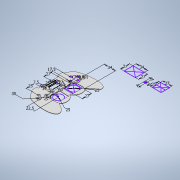
# Autodesk Inventor part: ovladac
Saved by Autodesk Inventor 2022 (Build 260153000, 153)
## iProperties
Created: 2022-12-02
Part Number: ovladac
Material: Generic
Document SubType Name: Modeling
Designer: matys
Density: 1 g/cm^3
Appearance: Default
Author: matys
Autodesk Inventor part; units mm, degrees
ref_plane "YZ Plane" through (0, 0, 0) normal (1, 0, 0) x (0, 1, 0)
ref_plane "XZ Plane" through (0, 0, 0) normal (0, 1, 0) x (-1, 0, 0)
ref_plane "XY Plane" through (0, 0, 0) normal (0, 0, 1) x (1, 0, 0)
sketch "Sketch1" plane through (0, 0, 0) normal (0, 1, 0) x (-1, 0, 0)
  circle A0 centre (0, 0) radius 17.5
  line L0 (0, -17.5) -> (0, -77.5)
  line L1 (0, -77.5) -> (0, -95)
  circle A1 centre (0, -95) radius 17.5
  line L2 (0, 0) -> (0, -25)
  line L3 (0, -25) -> (-22.5, -25)
  circle A2 centre (-22.5, -25) radius 12.5
  line L4 (-86.0476, -189.7218) -> (-86.0476, -216.7218)
  line L5 (-86.0476, -216.7218) -> (-52.0476, -216.7218)
  line L6 (-52.0476, -216.7218) -> (-52.0476, -189.7218)
  line L7 (-52.0476, -189.7218) -> (-86.0476, -189.7218)
  line L8 (-86.0476, -189.7218) -> (-52.0476, -216.7218)
  line L9 (-52.0476, -189.7218) -> (-86.0476, -216.7218)
  line L10 (0, -25) -> (0, -17.5)
  line L11 (0, -25) -> (0, -32.5)
  circle A3 centre (-22.5, -70) radius 12.5
  line L12 (-39.5, -56.5) -> (-39.5, -83.5)
  line L13 (-39.5, -83.5) -> (-5.5, -83.5)
  line L14 (-5.5, -83.5) -> (-5.5, -56.5)
  line L15 (-5.5, -56.5) -> (-39.5, -56.5)
  line L16 (-39.5, -56.5) -> (-5.5, -83.5)
  line L17 (-5.5, -56.5) -> (-39.5, -83.5)
  line L18 (-5.5, -56.5) -> (-22.5, -70)
  line L19 (-109.6323, -189.7218) -> (-115.6323, -189.7218)
  line L20 (-115.6323, -189.7218) -> (-115.6323, -195.7218)
  line L21 (-115.6323, -195.7218) -> (-109.6323, -195.7218)
  line L22 (-109.6323, -195.7218) -> (-109.6323, -189.7218)
  line L23 (-115.6323, -189.7218) -> (-109.6323, -195.7218)
  line L24 (-109.6323, -189.7218) -> (-115.6323, -195.7218)
  line L25 (0, -112.5) -> (0, -106)
  line L26 (-3, -109) -> (-3, -103)
  line L27 (-3, -103) -> (3, -103)
  line L28 (3, -103) -> (3, -109)
  line L29 (3, -109) -> (-3, -109)
  line L30 (14, -98) -> (8, -98)
  line L31 (14, -92) -> (14, -98)
  line L32 (8, -98) -> (8, -92)
  line L33 (8, -92) -> (14, -92)
  line L34 (3, -81) -> (3, -87)
  line L35 (-3, -81) -> (3, -81)
  line L36 (3, -87) -> (-3, -87)
  line L37 (-3, -87) -> (-3, -81)
  line L38 (-14, -92) -> (-8, -92)
  line L39 (-14, -98) -> (-14, -92)
  line L40 (-8, -92) -> (-8, -98)
  line L41 (-8, -98) -> (-14, -98)
  line L42 (-135.6088, -189.7218) -> (-135.6088, -214.7218)
  line L43 (-135.6088, -214.7218) -> (-162.6088, -214.7218)
  line L44 (-162.6088, -214.7218) -> (-162.6088, -189.7218)
  line L45 (-162.6088, -189.7218) -> (-135.6088, -189.7218)
  line L46 (-162.6088, -189.7218) -> (-135.6088, -214.7218)
  line L47 (-135.6088, -189.7218) -> (-162.6088, -214.7218)
  line L48 (17.5, 0) -> (17.5, -95)
  line L49 (-162.6088, -202.2218) -> (-135.6088, -202.2218)
  line L50 (25.5, -35) -> (25.5, -60)
  line L51 (25.5, -60) -> (-1.5, -60)
  line L52 (-1.5, -60) -> (-1.5, -35)
  line L53 (-1.5, -35) -> (25.5, -35)
  line L54 (25.5, -35) -> (20.5, -35)
  line L55 (20.5, -35) -> (20.5, -60)
  line L56 (-1.5, -35) -> (6.5, -35)
  line L57 (6.5, -35) -> (6.5, -60)
  line L58 (-1.5, -47.5) -> (6.5, -47.5)
  line L59 (-1.5, -35) -> (35.8, -35)
  line L60 (25.5, -60) -> (29.5, -60)
  line L61 (29.5, -60) -> (29.5, -47.5)
  line L62 (29.5, -47.5) -> (25.5, -47.5)
  line L63 (29.5, -60) -> (-7.8, -60)
  line L64 (-7.8, -60) -> (-7.8, -35)
  line L65 (-7.8, -35) -> (-1.5, -35)
  dimension "d0" = 35
  dimension "d1" = 60
  dimension "d2" = 17.5
  dimension "d3" = 25
  dimension "d4" = 22.5
  dimension "d6" = 25
  dimension "d7" = 27
  dimension "d8" = 34
  dimension "d9" = 27
  dimension "d10" = 7.5
  dimension "d11" = 25
  dimension "d12" = 27
  dimension "d13" = 34
  dimension "d14" = 27
  dimension "d15" = 6
  dimension "d16" = 6
  dimension "d17" = 6
  dimension "d18" = 6.5
  dimension "d22" = 6
  dimension "d25" = 360
  dimension "d27" = 25
  dimension "d28" = 27
  dimension "d32" = 25
  dimension "d33" = 27
  dimension "d34" = 5
  dimension "d35" = 8
  dimension "d36" = 8
  dimension "d72" = 37.3
  dimension "d73" = 4
  dimension "d74" = 37.3
  constraints: 132 end point, 20 perpendicular, 8 point on line, 8 vertical, 6 midpoint, 5 point on circle, 4 centre point, 3 coincident, 3 horizontal, 1 collinear, 1 tangent, 33 other
  measures "d0" diameter of A0
  measures "d1" distance of L0.start L0.end
  measures "d2" distance of L0.end L1.end
  measures "d3" distance of L2.start L2.end
  measures "d4" distance of L2.end L3.end
  measures "d6" diameter of A2
  measures "d7" distance of L4.start L4.end
  measures "d8" distance of L4.end L5.end
  measures "d9" distance of L5.end L6.end
  measures "d10" distance of L2.end L11.end
  measures "d11" diameter of A3
  measures "d12" distance of L15.end L12.end
  measures "d13" distance of L12.end L14.start
  measures "d14" distance of L14.start L15.start
  measures "d15" distance of L19.start L19.end
  measures "d16" distance of L19.end L20.end
  measures "d17" distance of L20.end L21.end
  measures "d18" distance of L25.start L25.end
  measures "d22" distance of L26.start L26.end
  measures "d27" distance of L42.start L42.end
  measures "d28" distance of L42.end L43.end
  measures "d32" distance of L50.start L50.end
  measures "d33" distance of L50.end L51.end
  measures "d34" distance of L50.start L54.end
  measures "d35" distance of L52.end L56.end
  measures "d36" distance between parallel lines of L50 L48
  measures "d72" distance of L52.end L59.end
  measures "d73" distance of L50.end L60.end
  measures "d74" distance of L60.end L63.end
sketch "Sketch2" plane through (0, 0, 0) normal (0, 1, 0) x (-1, 0, 0)
  circle A0 centre (0, 0) radius 17.5
  line L0 (0, 17.5) -> (0, 25.5)
  line L1 (17.5, 0) -> (29.5, 0)
  line L2 (0, 0) -> (0, 17.5)
  line L3 (0, 17.5) -> (17.5, 0)
  line L4 (0, 0) -> (8.75, 8.75)
  line L5 (8.75, 8.75) -> (12.3744, 12.3744)
  line L6 (12.3744, 12.3744) -> (18.0312, 18.0312)
  arc A1 (29.5, 0) -> (10.5727, 22.6518) centre (-3.4308, -8.2827) ccw
  line L7 (0, -20.5) -> (0, -80.5)
  line L8 (0, -80.5) -> (0, -98)
  line L9 (29.5, 0) -> (29.5, -17.5) construction
  line L10 (34.5, -12.5) -> (34.5, -5)
  arc A2 (34.5, -5) -> (29.5, 0) centre (29.5, -5) ccw
  arc A3 (29.5, -17.5) -> (34.5, -12.5) centre (29.5, -12.5) ccw
  line L11 (29.5, -17.5) -> (29.5, -47.5)
  line L12 (0, -20.5) -> (0, -25.5)
  line L13 (0, -17.5) -> (0, -21.5)
  ellipse E0 centre (-5.5218, 3.3783) end of major axis (-65.9225, 17.4065) minor radius 22.7978 (10.5727, 22.6518) -> (-28.0257, -13.7877) ccw
  line L14 (0, -17.5) -> (0, -25)
  line L15 (0, -25) -> (-22.5, -25)
  circle A4 centre (-22.5, -25) radius 12.5
  line L16 (-9, -8) -> (-36, -8)
  line L17 (-36, -8) -> (-36, -42)
  line L18 (-36, -42) -> (-9, -42)
  line L19 (-9, -42) -> (-9, -8)
  line L20 (-36, -42) -> (-9, -8)
  line L21 (-36, -8) -> (-9, -42)
  line L22 (-22.5, -25) -> (-36, -42)
  line L23 (0, -17.5) -> (0, -11)
  line L24 (0, -11) -> (3, -11)
  line L25 (3, -11) -> (3, -8)
  line L26 (3, -8) -> (-3, -8)
  line L27 (-3, -8) -> (-3, -14)
  line L28 (-3, -14) -> (3, -14)
  line L29 (3, -14) -> (3, -11)
  line L30 (14, 3) -> (11, 3)
  line L31 (8, 3) -> (8, -3)
  line L32 (11, 3) -> (8, 3)
  line L33 (8, -3) -> (14, -3)
  line L34 (14, -3) -> (14, 3)
  line L35 (-3, 14) -> (-3, 11)
  line L36 (-3, 8) -> (3, 8)
  line L37 (-3, 11) -> (-3, 8)
  line L38 (3, 8) -> (3, 14)
  line L39 (3, 14) -> (-3, 14)
  line L40 (-14, -3) -> (-11, -3)
  line L41 (-8, -3) -> (-8, 3)
  line L42 (-11, -3) -> (-8, -3)
  line L43 (-8, 3) -> (-14, 3)
  line L44 (-14, 3) -> (-14, -3)
  line L45 (0, -47.5) -> (-33.3972, -47.5)
  arc A5 (-41.1706, -8.3745) -> (-33.3972, -47.5) centre (-22.5, -25) ccw
  arc A6 (10.5727, -117.6518) -> (29.5, -95) centre (-3.4308, -86.7173) ccw
  line L46 (34.5, -82.5) -> (34.5, -90)
  arc A7 (29.5, -95) -> (34.5, -90) centre (29.5, -90) ccw
  arc A8 (34.5, -82.5) -> (29.5, -77.5) centre (29.5, -82.5) ccw
  line L47 (29.5, -77.5) -> (29.5, -47.5)
  ellipse E1 centre (-5.5218, -98.3783) end of major axis (-65.9225, -112.4065) minor radius 22.7978 (-28.0257, -81.2123) -> (10.5727, -117.6518) ccw
  arc A9 (-33.3972, -47.5) -> (-41.1706, -86.6255) centre (-22.5, -70) ccw
  line L48 (0, -95) -> (0, -112.5)
  line L49 (-9, -87) -> (-36, -87)
  line L50 (-36, -87) -> (-36, -53)
  line L51 (-36, -53) -> (-9, -53)
  line L52 (-9, -53) -> (-9, -87)
  line L53 (0, -77.5) -> (0, -84)
  line L54 (0, -84) -> (3, -84)
  line L55 (3, -84) -> (3, -87)
  line L56 (3, -87) -> (-3, -87)
  line L57 (-3, -87) -> (-3, -81)
  line L58 (-3, -81) -> (3, -81)
  line L59 (3, -81) -> (3, -84)
  line L60 (14, -98) -> (11, -98)
  line L61 (8, -98) -> (8, -92)
  line L62 (11, -98) -> (8, -98)
  line L63 (8, -92) -> (14, -92)
  line L64 (14, -92) -> (14, -98)
  line L65 (-3, -109) -> (-3, -106)
  line L66 (-3, -103) -> (3, -103)
  line L67 (-3, -106) -> (-3, -103)
  line L68 (3, -103) -> (3, -109)
  line L69 (3, -109) -> (-3, -109)
  line L70 (-14, -92) -> (-11, -92)
  line L71 (-8, -92) -> (-8, -98)
  line L72 (-11, -92) -> (-8, -92)
  line L73 (-8, -98) -> (-14, -98)
  line L74 (-14, -98) -> (-14, -92)
  line L75 (0, -47.5) -> (-1.5, -47.5)
  line L76 (-1.5, -47.5) -> (-1.5, -60)
  line L77 (-1.5, -60) -> (25.5, -60)
  line L78 (25.5, -60) -> (25.5, -35)
  line L79 (25.5, -35) -> (-1.5, -35)
  line L80 (-1.5, -35) -> (-1.5, -47.5)
  line L81 (0, -17.5) -> (0, -25)
  line L82 (0, -47.5) -> (0, -35)
  line L83 (25.5, -44.7664) -> (24.099, -44.7664)
  line L84 (-5.5218, 3.3783) -> (-65.9225, 17.4065)
  line L85 (-5.5218, 3.3783) -> (-5.5218, 9.5)
  line L86 (-65.9225, 17.4065) -> (128.8922, -27.8397)
  point P0 (29.5, -8.75)
  point P1 (0, -35)
  point P2 (0, -60)
  dimension "d50" = 25
  dimension "d37" = 35
  dimension "d38" = 8
  dimension "d39" = 12
  dimension "d40" = 8
  dimension "d41" = 60
  dimension "d42" = 17.5
  dimension "d47" = 4
  dimension "d48" = 7.5
  dimension "d49" = 22.5
  dimension "d51" = 27
  dimension "d52" = 34
  dimension "d53" = 6.5
  dimension "d54" = 3
  dimension "d55" = 3
  dimension "d56" = 6
  dimension "d57" = 6
  dimension "d60" = 360
  dimension "d65" = 1.5
  dimension "d66" = 12.5
  dimension "d67" = 27
  dimension "d68" = 25
  dimension "d69" = 1.401
  dimension "d70" = 76.925
  dimension "d71" = 200
  constraints: 176 end point, 41 symmetric about line, 25 point on circle, 22 point on line, 16 perpendicular, 9 centre point, 6 vertical, 4 horizontal, 3 coincident, 3 midpoint, 2 collinear, 2 tangent, 1 parallel, 61 other
  measures "d37" diameter of A0
  measures "d38" distance of L0.start L0.end
  measures "d39" distance of L1.end L1.start
  measures "d40" distance of L5.end L6.end
  measures "d41" distance of L7.start L7.end
  measures "d42" distance of L7.end L8.end
  measures "d47" distance of L13.start L13.end
  measures "d48" distance of L13.start L14.end
  measures "d49" distance of L14.end L15.end
  measures "d51" distance of L16.start L16.end
  measures "d52" distance of L16.end L17.end
  measures "d53" distance of L13.start L23.end
  measures "d54" distance of L23.end L24.end
  measures "d55" distance of L24.end L25.end
  measures "d56" distance of L25.end L26.end
  measures "d57" distance of L26.end L27.end
  measures "d65" distance of L45.start L75.end
  measures "d66" distance of L75.end L76.end
  measures "d67" distance of L76.end L77.end
  measures "d68" distance of L77.end L78.end
  measures "d69" distance of L83.start L83.end
  measures "d70" angle of L85 L84
  measures "d71" distance of L86.start L86.end
extrude "Extrusion1" add sketch "Sketch2" along normal blind 1 contours L3 L5 A0 | L1 A2 L10 L86 A0 | A0 L6 A1 L1 | A0 L86 L34 L30 L32 L31 L4 L3 | L5 L3 A0 | A0 L0 E0 A1 L6 | L86 L10 A3 L11 L47 A8 L46 A7 A6 E1 A9 L45 L76 L77 L78 L79 L7 L13 A0 | A0 L19 L16 L84 L86 L2 L4 L31 L33 L34 | L4 L86 L2 L36 L38 L39 L3 | L2 L39 L35 L37 L36 L86 L84 A0 | A0 L84 E0 L0 | L13 L7 L15 L19 A0 | L4 L2 L86 | A0 L16 L17 E0 L84 | L15 L7 L79 L80 L45 A5 E0 L17 L18 L19 | L80 L79 L7 L45 | L45 L7 L77 L76
body "Solid1"
